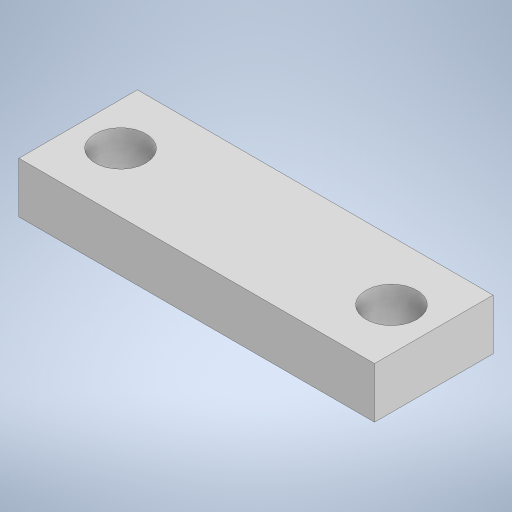
# Autodesk Inventor part: linear rod support mount spacer
Saved by Autodesk Inventor 2023.2 (Build 272271000, 271)
## iProperties
Created: 2023-03-17
Part Number: linear rod support mount spacer
Material: Generic
Document SubType Name: Modeling
Designer: dmargari
Density: 1 g/cm^3
Appearance: Default
Author: dmargari
## iProperties of the stored document linear rod support mount spacer_3DPrint.ipt
Created: 2023-03-17
Part Number: linear rod support mount spacer_3DPrint
Material: Generic
Document SubType Name: Modeling
Designer: dmargari
Density: 1 g/cm^3
Appearance: Default
Author: dmargari
Autodesk Inventor part; units mm, degrees
ref_plane "YZ Plane" through (0, 0, 0) normal (1, 0, 0) x (0, 1, 0)
ref_plane "XZ Plane" through (0, 0, 0) normal (0, 1, 0) x (-1, 0, 0)
ref_plane "XY Plane" through (0, 0, 0) normal (0, 0, 1) x (1, 0, 0)
sketch "Sketch1" plane through (0, 0, 0) normal (0, 1, 0) x (-1, 0, 0)
  line L0 (59.7159, -8.8837) -> (17.7159, -8.8837)
  line L1 (17.7159, -8.8837) -> (17.7159, -22.8837)
  line L2 (17.7159, -22.8837) -> (59.7159, -22.8837)
  line L3 (59.7159, -22.8837) -> (59.7159, -8.8837)
  line L4 (59.7159, -8.8837) -> (17.7159, -22.8837) construction
  line L5 (17.7159, -8.8837) -> (59.7159, -22.8837) construction
  line L6 (59.7159, -15.8837) -> (17.7159, -15.8837) construction
  point P0 (0, 0)
  point P1 (38.7159, -15.8837)
  point P2 (54.7159, -15.8837)
  point P3 (22.7159, -15.8837)
  dimension "d0" = 42
  dimension "d1" = 14
  dimension "d2" = 5
  dimension "d3" = 5
  constraints: 14 end point, 4 midpoint, 2 parallel, 2 point on line, 1 horizontal, 1 perpendicular
  measures "d0" distance of L2.end L1.end
  measures "d1" distance of L1.end L0.end
  measures "d2" distance from line of L3 point (54.716, -15.884)
  measures "d3" distance from line of L1 point (22.716, -15.884)
extrude "Extrusion1" add sketch "Sketch1" along normal blind 6
hole "Hole1" at (-54.7159, 0, -15.8837) at (-22.7159, 0, -15.8837) direction (0, 1, 0) diameter 6 end through all
body "Solid1"
